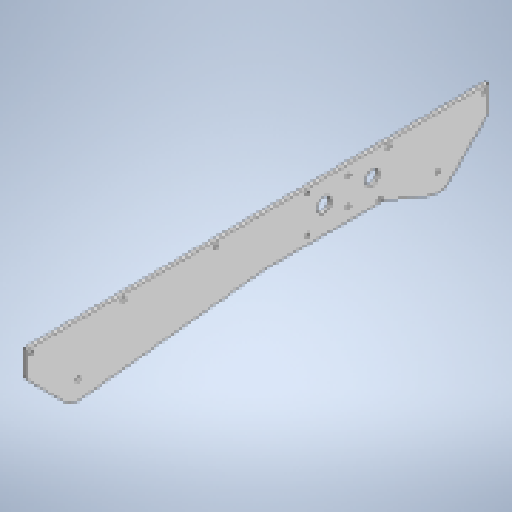
# Autodesk Inventor part: Outside Chassi Plate
Saved by Autodesk Inventor 2023 (Build 270158000, 158)
## iProperties
Created: 2022-09-05
Part Number: Outside Chassi Plate
Material: Generic
Document SubType Name: Modeling
Designer: deli
Density: 1 g/cm^3
Appearance: Default
Author: deli
Autodesk Inventor part; units mm, degrees
ref_plane "YZ Plane" through (0, 0, 0) normal (1, 0, 0) x (0, 1, 0)
ref_plane "XZ Plane" through (0, 0, 0) normal (0, 1, 0) x (-1, 0, 0)
ref_plane "XY Plane" through (0, 0, 0) normal (0, 0, 1) x (1, 0, 0)
sketch "Sketch1" plane through (0, 0, 0) normal (1, 0, 0) x (0, 1, 0)
  line L0 (-206.1359, 514.9611) -> (-206.1359, 64.9611)
  line L1 (-206.1359, 514.9611) -> (-231.1359, 514.9611)
  line L2 (-231.1359, 514.9611) -> (-268.7861, 477.7662)
  line L3 (-206.1359, 64.9611) -> (-231.1359, 64.9611)
  line L4 (-231.1359, 64.9611) -> (-268.7861, 102.1559)
  line L5 (-272.6687, 122.0791) -> (-254.1359, 165.1245)
  line L6 (-254.1359, 165.1245) -> (-254.1359, 299.8441)
  line L7 (-254.1359, 299.8441) -> (-274.0035, 462.7824)
  circle A0 centre (-256.1359, 464.9611) radius 2
  arc A1 (-268.7861, 477.7662) -> (-274.0035, 462.7824) centre (-256.1359, 464.9611) ccw
  circle A2 centre (-256.1359, 464.9611) radius 48 construction
  arc A3 (-244.2968, 466.484) -> (-267.9847, 463.5163) centre (-256.1359, 464.9611) ccw construction
  circle A4 centre (-256.1359, 114.9611) radius 48 construction
  arc A5 (-267.0995, 119.6814) -> (-245.2762, 110.0061) centre (-256.1359, 114.9611) ccw construction
  arc A6 (-272.6687, 122.0791) -> (-268.7861, 102.1559) centre (-256.1359, 114.9611) ccw
  circle A7 centre (-256.1359, 114.9611) radius 2
  circle A8 centre (-226.1359, 225.5003) radius 7
  circle A9 centre (-226.1359, 182.6285) radius 7
  circle A10 centre (-226.1359, 225.5003) radius 16 construction
  circle A11 centre (-226.1359, 182.6285) radius 16 construction
  arc A12 (-238.7746, 223.9592) -> (-213.5075, 227.1247) centre (-226.1359, 225.5003) ccw construction
  arc A13 (-214.5523, 177.3433) -> (-237.8304, 187.6635) centre (-226.1359, 182.6285) ccw construction
  line L8 (-244.2968, 466.484) -> (-213.5075, 227.1247) construction
  line L9 (-238.7746, 223.9592) -> (-267.9847, 463.5163) construction
  line L10 (-214.5523, 177.3433) -> (-245.2762, 110.0061) construction
  line L11 (-267.0995, 119.6814) -> (-237.8304, 187.6635) construction
  circle A14 centre (-214.1359, 242.1211) radius 2
  circle A15 centre (-215.3422, 204.0644) radius 2
  circle A16 centre (-236.9295, 204.0644) radius 2
  circle A17 centre (-246.1359, 230.0003) radius 2
  circle A18 centre (-246.1359, 178.1285) radius 2
  circle A19 centre (-214.1359, 166.0078) radius 2
  circle A20 centre (-211.1359, 509.9611) radius 2
  circle A21 centre (-211.1359, 69.9611) radius 2
  circle A22 centre (-211.1359, 420.6755) radius 2
  circle A23 centre (-211.1359, 331.3899) radius 2
  point P0 (0, 0)
  dimension "d43" = 450
  dimension "d44" = 4
  dimension "d45" = 36
  dimension "d46" = 96
  dimension "d47" = 23.8732
  dimension "d48" = 96
  dimension "d49" = 4
  dimension "d50" = 36
  dimension "d51" = 23.8732
  dimension "d52" = 50
  dimension "d53" = 50
  dimension "d54" = 50
  dimension "d55" = 50
  dimension "d56" = 25
  dimension "d57" = 25
  dimension "d58" = 14
  dimension "d59" = 14
  dimension "d60" = 32
  dimension "d61" = 32
  dimension "d62" = 25.4648
  dimension "d63" = 25.4648
  dimension "d64" = 179.622
  dimension "d65" = 179.622
  dimension "d66" = 178.768
  dimension "d67" = 178.768
  dimension "d68" = 241.3313
  dimension "d69" = 20
  dimension "d70" = 74.0152
  dimension "d71" = 20
  dimension "d72" = 48
  dimension "d73" = 4
  dimension "d74" = 4
  dimension "d75" = 4
  dimension "d77" = 4
  dimension "d78" = 4
  dimension "d90" = 6
  dimension "d91" = 6
  dimension "d92" = 6
  dimension "d93" = 6
  dimension "d94" = 2.5
  dimension "d95" = 2.5
  dimension "d96" = 2.5
  dimension "d97" = 2.5
  dimension "d98" = 8
  dimension "d99" = 8
  dimension "d100" = 117.444
  dimension "d103" = 4
  dimension "d104" = 4
  dimension "d105" = 4
  dimension "d106" = 4
  dimension "d107" = 5
  dimension "d108" = 5
  dimension "d109" = 5
  dimension "d110" = 5
  dimension "d111" = 5
  dimension "d112" = 5
  dimension "d113" = 267.8568
  dimension "d114" = 89.2856
  dimension "d115" = 89.2856
  dimension "d118" = 8
  dimension "d119" = 8
  dimension "d120" = 4
  constraints: 24 centre point, 24 end point, 12 point on circle, 12 tangent, 10 coincident, 2 parallel, 2 perpendicular, 2 vertical
  measures "d43" distance of L0.start L0.end
  measures "d44" diameter of A0
  measures "d45" diameter of A1
  measures "d46" diameter of A2
  measures "d47" diameter of A3
  measures "d48" diameter of A4
  measures "d49" diameter of A7
  measures "d50" diameter of A6
  measures "d51" diameter of A5
  measures "d52" distance from line of L0 A1.centre
  measures "d53" distance from line of L0 A4.centre
  measures "d54" distance from line of A0.centre L1
  measures "d55" distance from line of L3 A7.centre
  measures "d56" distance of L0.start L1.end
  measures "d57" distance of L0.end L3.end
  measures "d58" diameter of A8
  measures "d59" diameter of A9
  measures "d60" diameter of A10
  measures "d61" diameter of A11
  measures "d62" diameter of A12
  measures "d63" diameter of A13
  measures "d68" distance of L8.start L8.end
  measures "d69" distance from line of L0 A8.centre
  measures "d70" distance of L10.start L10.end
  measures "d71" distance from line of L0 A9.centre
  measures "d72" distance between parallel lines of L0 L6
  measures "d73" diameter of A14
  measures "d74" diameter of A17
  measures "d75" diameter of A16
  measures "d77" diameter of A15
  measures "d78" diameter of A19
  measures "d98" distance from line of L0 A14.centre
  measures "d99" distance from line of L0 A19.centre
  measures "d103" diameter of A20
  measures "d104" diameter of A22
  measures "d105" diameter of A23
  measures "d106" diameter of A21
  measures "d107" distance from line of L0 A20.centre
  measures "d108" distance from line of L1 A20.centre
  measures "d109" distance from line of L0 A22.centre
  measures "d110" distance from line of L0 A23.centre
  measures "d111" distance from line of L0 A21.centre
  measures "d112" distance from line of L3 A21.centre
  measures "d113" distance of A14.centre A20.centre
  measures "d114" distance of A22.centre A20.centre
  measures "d115" distance of A23.centre A22.centre
  measures "d118" distance from line of L6 A18.centre
  measures "d119" distance from line of L6 A17.centre
  measures "d120" diameter of A18
extrude "Extrusion1" add sketch "Sketch1" along normal blind 3.175
body "Solid1"
